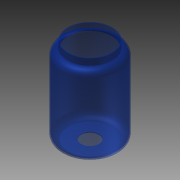
# Autodesk Inventor part: Vessel
Saved by Autodesk Inventor 2011 (Build 150239000, 239)
## iProperties
Created: 2013-10-24
Part Number: Vessel
Document SubType Name: Modeling
Designer: Devon
Density: 1 g/cm^3
Author: Devon
Autodesk Inventor part; units mm, degrees
ref_plane "YZ Plane" through (0, 0, 0) normal (1, 0, 0) x (0, 1, 0)
ref_plane "XZ Plane" through (0, 0, 0) normal (0, 1, 0) x (-1, 0, 0)
ref_plane "XY Plane" through (0, 0, 0) normal (0, 0, 1) x (1, 0, 0)
sketch "Sketch1" plane through (0, 0, 0) normal (0, 0, 1) x (1, 0, 0)
  line L0 (0, 0) -> (0, 1.5875)
  line L1 (0, 0) -> (0, 1.5875)
  line L2 (17.4625, 1.5875) -> (17.4625, 0)
  line L3 (17.4625, 0) -> (44.4373, 0)
  line L4 (57.1373, 12.7) -> (57.1373, 146.05)
  line L5 (55.5498, 144.4625) -> (55.5498, 14.2875)
  line L6 (17.4625, 1.5875) -> (42.8498, 1.5875)
  arc A0 (44.4373, 0) -> (57.1373, 12.7) centre (44.4373, 12.7) ccw
  arc A1 (42.8498, 1.5875) -> (55.5498, 14.2875) centre (42.8498, 14.2875) ccw
  line L7 (42.8498, 157.1625) -> (42.8498, 158.75)
  line L8 (42.8498, 158.75) -> (44.4373, 158.75)
  line L9 (42.8498, 158.75) -> (42.8498, 157.1625)
  line L10 (42.8498, 157.1625) -> (42.8498, 157.1625)
  arc A2 (55.5498, 144.4625) -> (42.8498, 157.1625) centre (42.8498, 144.4625) ccw
  arc A3 (57.1373, 146.05) -> (44.4373, 158.75) centre (44.4373, 146.05) ccw
  line L11 (42.8498, 157.1625) -> (41.2623, 157.1625)
  line L12 (42.8498, 158.75) -> (42.8498, 171.45)
  line L13 (42.8498, 171.45) -> (41.2623, 171.45)
  line L14 (41.2623, 171.45) -> (41.2623, 157.1625)
  point P0 (57.1373, 0)
  dimension "d4" = 1.5875
  dimension "d5" = 17.4625
  dimension "d10" = 39.6748
  dimension "d14" = 12.7
  dimension "d15" = 1.5875
  dimension "d16" = 12.7
  dimension "d17" = 1.5875
  dimension "d18" = 12.7
  constraints: 30 end point, 9 perpendicular, 9 tangent, 8 point on circle, 4 centre point, 2 equal radius, 2 point on line, 1 parallel
  measures "d4" distance of L0.start L0.end
  measures "d5" distance of L0.end L2.start
  measures "d10" distance of L2.end point (57.137, 0)
  measures "d14" radius of A0
  measures "d15" distance of L7.end L7.start
  measures "d16" radius of A2
  measures "d17" distance of L10.end L11.end
  measures "d18" distance of L7.end L12.end
revolve "Revolution1" add sketch "Sketch1" angle 360 about axis through (0, 0, 0) along (0, 1, 0) contours L6 A1 L5 A2 L7 L8 A3 L4 A0 L3 L2
sketch "Sketch2" plane through (0, 50.8, 0) normal (0, 1, 0) x (1, 0, 0)
  circle A0 centre (0, 0) radius 69.85 projected
  circle A1 centre (0, 0) radius 68.2625 projected
  circle A2 centre (0, 0) radius 68.2625
  circle A3 centre (0, 0) radius 69.85
  constraints: 2 centre point, 2 coincident, 2 concentric
extrude "Extrusion1" [suppressed]
sketch "Sketch3" plane through (0, 158.75, 0) normal (0, 1, 0) x (1, 0, 0)
  circle A0 centre (0, 0) radius 44.4373 projected
  circle A1 centre (0, 0) radius 42.8498 projected
  circle A2 centre (0, 0) radius 42.8498
  circle A3 centre (0, 0) radius 44.4373
  constraints: 2 centre point, 2 coincident, 2 concentric
extrude "Extrusion2" add sketch "Sketch3" along normal blind 12.7
body "Solid1"
